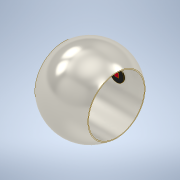
# Autodesk Inventor part: Smart Ring
Saved by Autodesk Inventor 2020 (Build 240168000, 168)
## iProperties
Created: 2020-05-02
Part Number: Smart Ring
Material: Titanium
Document SubType Name: Modeling
Designer: harry
Density: 4.51 g/cm^3
Appearance: Titanium
Author: harry
Autodesk Inventor part; units mm, degrees
ref_plane "YZ Plane" through (0, 0, 0) normal (1, 0, 0) x (0, 1, 0)
ref_plane "XZ Plane" through (0, 0, 0) normal (0, 1, 0) x (-1, 0, 0)
sketch "Sketch1" plane through (0, 0, 0) normal (0, 1, 0) x (-1, 0, 0)
  line L0 (9.5, 0) -> (-9.5, 0)
  line L1 (9.5, 0) -> (9.5, -10) construction
  line L2 (-9.5, 0) -> (-9.5, -10) construction
  line L3 (9.5, -10) -> (9.5, -10.2835)
  line L4 (-9.5, -10) -> (-9.5, -10.2835)
  arc A0 (-9.5, -10.2835) -> (9.5, -10.2835) centre (0, 0) ccw
  line L5 (9.5, -10) -> (-9.5, -10)
  dimension "d0" = 19
  dimension "d7" = 14
  dimension "d9" = 10
  constraints: 12 end point, 4 vertical, 3 coincident, 2 horizontal, 2 parallel, 2 point on circle, 1 centre point, 1 midpoint
  measures "d0" distance of L0.start L0.end
  measures "d7" radius of A0
  measures "d9" distance from line of L5 point (0, 0)
ref_plane "Work Plane1" through (0, 0, -10) normal (0, 0, 1) x (1, 0, 0)
revolve "Revolution2" add sketch "Sketch1" angle 360 about axis through (-9.5, 0, 0) along (1, 0, 0)
sketch "Sketch4" plane through (0, 0, -10) normal (0, 0, 1) x (1, 0, 0)
  circle A0 centre (0, 0) radius 2.5
  dimension "d17" = 5
  constraints: 1 centre point, 1 coincident
  measures "d17" diameter of A0
extrude "Extrusion3" add sketch "Sketch4" along normal blind 0.4
sketch "Sketch5" plane through (0, 0, -9.6) normal (0, 0, 1) x (1, 0, 0)
  circle A0 centre (0, 0) radius 2.5 projected
  line L0 (0.75, 0.75) -> (0.75, -0.75)
  line L1 (0.75, -0.75) -> (-0.75, -0.75)
  line L2 (-0.75, -0.75) -> (-0.75, 0.75)
  line L3 (-0.75, 0.75) -> (0.75, 0.75)
  point P0 (0.5831, -2.431)
  point P1 (0.5831, 2.431)
  dimension "d20" = 1.5
  constraints: 8 end point, 1 coincident, 1 horizontal, 9 other
  measures "d20" distance of L2.end L0.start
extrude "Extrusion4" add sketch "Sketch5" along normal blind 0.1 contours L0 L1 L2 L3
body "Solid2"
